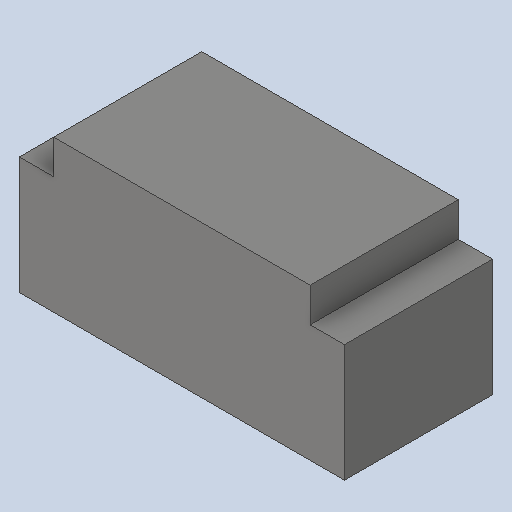
# Autodesk Inventor part: GUS Zentriereinsatz
Saved by Autodesk Inventor 2023 (Build 270158000, 158)
## iProperties
Created: 2023-08-22
Part Number: GUS Zentriereinsatz
Material: Generic
Catalog Web Link: www.cadenas.de
Description: GUS Zentriereinsatz-Zentriereinsatz
Vendor: ROBOTUNITS
Document SubType Name: Modeling
Designer: psAdmin
Manufacturer: ROBOTUNITS
Mass: 1.18064 g
Surface Area: 7.2092 cm^2
Volume: 1.18064 cm^3
Density: 1 g/cm^3
Appearance: PSOLRGB-128-128-128
Category: PARTsolutions
Company: ROBOTUNITS
PSOL_IDENT_0: {$CADENAS_DATA/23d-libs/robotunits/profil_und_verbindungstechnik/verbindungstechnik_raster_40/parts/
PSOL_IDENT_1: zentriereinsatz.prj},191 {VTYP=3D},{NB=GUS Zentriereinsatz},{LINA=GUS Zentriereinsatz},{NN=GUS Zentr
PSOL_IDENT_2: iereinsatz},{DATE=25.04.2023 11:21:45},{GEOMDATE=05.01.2012 13:55:00},{VERSION=},{LINEID=10},{WBVAR=
PSOL_IDENT_3: },{WBNUMERIC=}  {NB=GUS Zentriereinsatz},{LINA=GUS Zentriereinsatz},{KT=DUMMY},{IDNR=},{L=18.000},{B=
PSOL_IDENT_4: 8.400}
NB: GUS Zentriereinsatz
NN: GUS Zentriereinsatz
NT: Zentriereinsatz
NBSYN: GUS Zentriereinsatz
LINA: GUS Zentriereinsatz
CATALOG: Robotunits
L: 18
B: 8.4
SUPPLIER: ROBOTUNITS
ARTICLENO: GUS Zentriereinsatz
BOMINFO: GUS Zentriereinsatz
CREATOR: CADENAS GmbH
Title: GUS Zentriereinsatz
Author: Cadenas PARTsolutions
Comments: Zentriereinsatz
Autodesk Inventor part; units mm, degrees
sketch "Sketch_1" plane through (0, 0, 0) normal (0, 0, 1) x (1, 0, 0)
  line L0 (-9, 6.5) -> (-9, 0)
  line L1 (-9, 0) -> (9, 0)
  line L2 (9, 0) -> (9, 6.5)
  line L3 (9, 6.5) -> (7.1, 6.5)
  line L4 (7.1, 6.5) -> (7.1, 8.4)
  line L5 (7.1, 8.4) -> (-7.1, 8.4)
  line L6 (-7.1, 8.4) -> (-7.1, 6.5)
  line L7 (-7.1, 6.5) -> (-9, 6.5)
  constraints: 16 end point
extrude "Extrusion1" add sketch "Sketch_1" along normal mid plane 8.2
ref_plane "p1_XY" through (0, 0, 0) normal (0, 1, 0) x (1, 0, 0)
ref_plane "p1_YZ" through (0, 0, 0) normal (1, 0, 0) x (0, 0, -1)
ref_plane "p1_ZX" through (0, 0, 0) normal (0, 0, -1) x (0, 1, 0)
body "Solid1"
